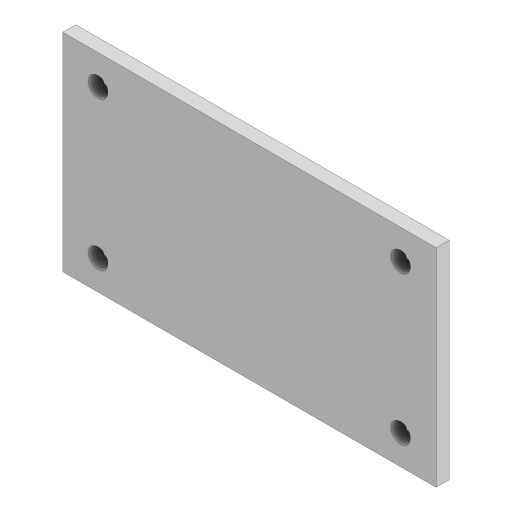
# Autodesk Inventor part: baseplate
Saved by Autodesk Inventor 2024 (Build 280153000, 153)
## iProperties
Created: 2024-01-27
Part Number: baseplate
Material: Generic
Document SubType Name: Modeling
Designer: chris
Density: 1 g/cm^3
Appearance: Default
Author: chris
Autodesk Inventor part; units mm, degrees
ref_plane "YZ Plane" through (0, 0, 0) normal (1, 0, 0) x (0, 1, 0)
ref_plane "XZ Plane" through (0, 0, 0) normal (0, 1, 0) x (-1, 0, 0)
ref_plane "XY Plane" through (0, 0, 0) normal (0, 0, 1) x (1, 0, 0)
sketch "Sketch1" plane through (0, 0, 0) normal (0, 0, 1) x (1, 0, 0)
  line L0 (0, 0) -> (0, 50.8)
  line L1 (0, 50.8) -> (76.2, 50.8)
  line L2 (76.2, 50.8) -> (76.2, 0)
  line L3 (76.2, 0) -> (0, 0)
  circle A0 centre (61.2521, 14.0462) radius 1.5
  circle A1 centre (14.9479, 14.0462) radius 1.5
  circle A2 centre (61.2521, 36.7538) radius 1.5
  circle A3 centre (14.9479, 36.7538) radius 1.5
  line L4 (14.9479, 36.7538) -> (14.9479, 14.0462)
  line L5 (0, 25.4) -> (-9.2458, 25.4)
  line L6 (66.675, 41.275) -> (9.525, 41.275)
  line L7 (9.525, 41.275) -> (9.525, 9.525)
  line L8 (9.525, 9.525) -> (66.675, 9.525)
  line L9 (66.675, 9.525) -> (66.675, 41.275)
  dimension "d0" = 50.8
  dimension "d1" = 76.2
  dimension "d2" = 3
  dimension "d3" = 3
  dimension "d4" = 9.525
  constraints: 20 end point, 4 centre point, 4 perpendicular, 2 horizontal, 2 vertical, 1 midpoint, 3 other
  measures "d0" distance of L0.start L0.end
  measures "d1" distance of L0.end L1.end
  measures "d2" diameter of A2
  measures "d3" diameter of A0
  measures "d4" distance between parallel lines of L1 L6
extrude "Extrusion1" add sketch "Sketch1" along normal blind 2 contours L9 L8 L7 L6
body "Solid1"
